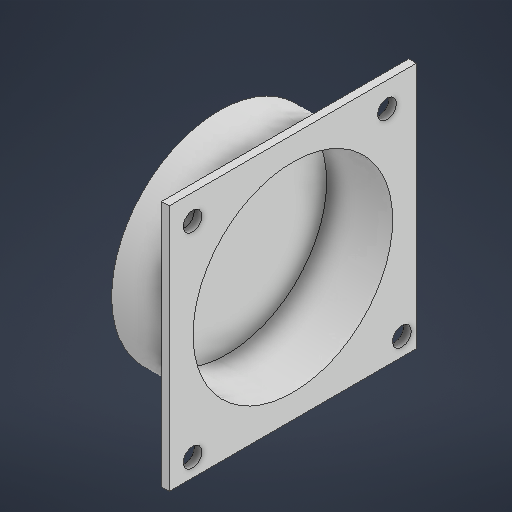
# Autodesk Inventor part: MagnetCap
Saved by Autodesk Inventor 2027 (Build 310192000, 192)
## iProperties
Created: 2026-06-10
Part Number: MagnetCap
Material: Generic
Document SubType Name: Modeling
Designer: giese
Density: 1 g/cm^3
Appearance: Default
Author: giese
Autodesk Inventor part; units mm, degrees
ref_plane "YZ Plane" through (0, 0, 0) normal (1, 0, 0) x (0, 1, 0)
ref_plane "XZ Plane" through (0, 0, 0) normal (0, 1, 0) x (-1, 0, 0)
ref_plane "XY Plane" through (0, 0, 0) normal (0, 0, 1) x (1, 0, 0)
sketch "Sketch1" plane through (0, 0, 0) normal (1, 0, 0) x (0, 1, 0)
  circle A0 centre (0, 0) radius 17.78
  dimension "d0" = 35.56
  constraints: 1 centre point, 1 coincident
  measures "d0" diameter of A0
extrude "Extrusion1" add sketch "Sketch1" along normal blind 1.27
sketch "Sketch2" plane through (1.27, 0, 0) normal (1, 0, 0) x (0, 0, -1)
  circle A0 centre (0, 0) radius 17.78
  circle A1 centre (0, 0) radius 16.51
  dimension "d3" = 35.56
  dimension "d4" = 33.02
  constraints: 2 centre point, 2 coincident
  measures "d3" diameter of A0
  measures "d4" diameter of A1
extrude "Extrusion2" add sketch "Sketch2" along normal blind 9.652
sketch "Sketch3" plane through (10.922, 0, 0) normal (1, 0, 0) x (0, 0, -1)
  line L0 (-20.45, -20.45) -> (20.45, -20.45)
  line L1 (20.45, -20.45) -> (20.45, 20.45)
  line L2 (20.45, 20.45) -> (-20.45, 20.45)
  line L3 (-20.45, 20.45) -> (-20.45, -20.45)
  line L4 (-20.45, -20.45) -> (20.45, 20.45) construction
  line L5 (20.45, -20.45) -> (-20.45, 20.45) construction
  point P0 (0, 0)
  dimension "d7" = 40.9
  dimension "d8" = 40.9
  constraints: 12 end point, 2 midpoint, 2 parallel, 1 horizontal, 1 perpendicular
  measures "d7" distance between parallel lines of L0 L2
  measures "d8" distance between parallel lines of L1 L3
extrude "Extrusion3" add sketch "Sketch3" along normal blind 1.27
sketch "Sketch4" plane through (12.192, 0, 0) normal (1, 0, 0) x (0, 0, -1)
  circle A0 centre (-16.5903, 16.3218) radius 1.55
  circle A1 centre (-16.5903, -17.4782) radius 1.55
  circle A2 centre (15.5877, 16.3218) radius 1.55
  circle A3 centre (18.0371, -17.4782) radius 1.55
  circle A4 centre (0, 0) radius 16.51
  dimension "d11" = 33.8
  dimension "d12" = 3.1
  dimension "d13" = 3.1
  dimension "d14" = 3.1
  dimension "d15" = 3.1
  dimension "d18" = 33.02
  constraints: 5 centre point, 1 coincident
  measures "d11" distance of A1.centre A0.centre
  measures "d12" diameter of A0
  measures "d13" diameter of A1
  measures "d14" diameter of A2
  measures "d15" diameter of A3
  measures "d18" diameter of A4
extrude "Extrusion4" cut sketch "Sketch4" against normal blind 1.27
fillet "Fillet1" radius 1.778 1 edges at (10.922, 0, 17.78)
sketch "Sketch5" plane through (0, 0, 0) normal (-1, 0, 0) x (0, 0, 1)
  point P0 (0, 0)
body "Solid1"
